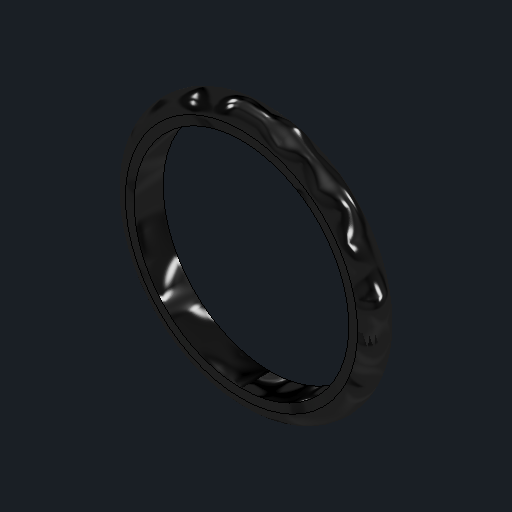
# Autodesk Inventor part: 36mm tamiya-slim-tire-gomu
Saved by Autodesk Inventor 2023.2 (Build 272271030, 271C)
## iProperties
Created: 2023-10-14
Part Number: 36mm tamiya-slim-tire-gomu
Material: ABS Plastic
Document SubType Name: Modeling
Designer: takag
Density: 1.06 g/cm^3
Appearance: 黒
Mass: 1.1974 g
Surface Area: 12.8611 cm^2
Volume: 1.12962 cm^3
Author: takag
Autodesk Inventor part; units mm, degrees
ref_plane "YZ Plane" through (0, 0, 0) normal (1, 0, 0) x (0, 1, 0)
ref_plane "XZ Plane" through (0, 0, 0) normal (0, 1, 0) x (-1, 0, 0)
ref_plane "XY Plane" through (0, 0, 0) normal (0, 0, 1) x (1, 0, 0)
sketch "スケッチ1" plane through (0, 0, 0) normal (1, 0, 0) x (0, 1, 0)
  line L0 (14.8, 0) -> (14.8, 2)
  line L1 (14.8, 0) -> (14.8, -2)
  circle A0 centre (16, 0) radius 2
  line L2 (14.8, 2) -> (16, 2)
  line L3 (14.8, -2) -> (16, -2)
  line L4 (0, 0) -> (0, -5)
  point P0 (18, 0)
  dimension "d0" = 2
  dimension "d1" = 2
  dimension "d3" = 18
  dimension "d4" = 4
  dimension "d5" = 5
  dimension "d7" = 3.2
  constraints: 10 end point, 3 point on circle, 3 vertical, 2 horizontal alignment, 2 tangent, 1 centre point, 1 horizontal
  measures "d0" distance of L0.start L0.end
  measures "d1" distance of L0.start L1.end
  measures "d3" distance of L4.start A0.start
  measures "d4" diameter of A0
  measures "d5" distance of L4.start L4.end
revolve "回転1" add sketch "スケッチ1" angle 360 about axis through (0, 0, 0) along (0, 0, -1) picked at (16.9166, -0.1483) contours L0 A0 L1 | L0 L2 A0 | A0 L3 L1
